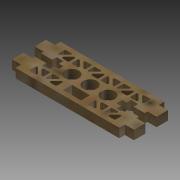
# Autodesk Inventor part: MotorCableHolder
Saved by Autodesk Inventor 2012 (Build 160160000, 160)
## iProperties
Created: 2014-07-20
Part Number: MotorCableHolder
Material: Default
Document SubType Name: Modeling
Designer: Anon
Density: 1 g/cm^3
Author: Anon
Autodesk Inventor part; units mm, degrees
ref_plane "YZ Plane" through (0, 0, 0) normal (1, 0, 0) x (0, 1, 0)
ref_plane "XZ Plane" through (0, 0, 0) normal (0, 1, 0) x (-1, 0, 0)
sketch "Sketch1" plane through (0, 0, 0) normal (0, 0, 1) x (1, 0, 0)
  line L0 (-27, 7.5) -> (-27, 2.5)
  line L1 (-27, 2.5) -> (-23, 2.5)
  line L2 (-27, 7.5) -> (-23, 7.5)
  line L3 (-23, 7.5) -> (-23, 10)
  line L4 (-23, 10) -> (0, 10)
  line L5 (0, 10) -> (0, 0)
  line L6 (0, 0) -> (-23, 0)
  line L7 (-23, 2.5) -> (-23, 0)
  line L8 (-27, -7.5) -> (-27, -2.5)
  line L9 (-27, -2.5) -> (-23, -2.5)
  line L10 (-27, -7.5) -> (-23, -7.5)
  line L11 (-23, -7.5) -> (-23, -10)
  line L12 (-23, -10) -> (0, -10)
  line L13 (0, -10) -> (0, 0)
  line L14 (-23, -2.5) -> (-23, 0)
  line L15 (27, 7.5) -> (27, 2.5)
  line L16 (27, 2.5) -> (23, 2.5)
  line L17 (27, 7.5) -> (23, 7.5)
  line L18 (23, 7.5) -> (23, 10)
  line L19 (23, 10) -> (0, 10)
  line L20 (0, 0) -> (23, 0)
  line L21 (23, 2.5) -> (23, 0)
  line L22 (27, -7.5) -> (27, -2.5)
  line L23 (27, -2.5) -> (23, -2.5)
  line L24 (27, -7.5) -> (23, -7.5)
  line L25 (23, -7.5) -> (23, -10)
  line L26 (23, -10) -> (0, -10)
  line L27 (23, -2.5) -> (23, 0)
  dimension "d0" = 5
  dimension "d1" = 4
  dimension "d12" = 27
  dimension "d13" = 4
  dimension "d14" = 2.5
  dimension "d53" = 2.5
  constraints: 56 end point, 17 symmetric about line, 3 perpendicular, 2 parallel, 1 vertical
  measures "d0" distance of L0.start L0.end
  measures "d1" distance of L0.end L1.end
  measures "d12" distance from line of L5.end L0
  measures "d13" distance of L0.start L2.end
  measures "d14" distance of L2.end L3.end
  measures "d53" distance of L1.end L6.end
extrude "Base" add sketch "Sketch1" along normal blind 4
sketch "Sketch2" plane through (0, 0, 4) normal (0, 0, 1) x (1, 0, 0)
  line L0 (-23, -2.5) -> (-23, 2.5) projected
  line L1 (-23, -10) -> (-23, -7.5) projected
  line L2 (-23, 1.25) -> (-18, 1.25)
  line L3 (-18, 1.25) -> (-18, 3.25)
  line L4 (-18, 3.25) -> (-15, 3.25)
  line L5 (-15, 3.25) -> (-15, 1.25)
  line L6 (-15, 1.25) -> (-13, 1.25)
  line L7 (-13, 1.25) -> (-13, -1.25)
  line L8 (-13, -1.25) -> (-15, -1.25)
  line L9 (-15, -1.25) -> (-15, -3.25)
  line L10 (-15, -3.25) -> (-18, -3.25)
  line L11 (-18, -3.25) -> (-18, -1.3408)
  line L12 (-18, -1.3408) -> (-23, -1.3408)
  line L13 (-23, 1.25) -> (-23, -1.3408)
  point P0 (0, 0)
  dimension "d17" = 5
  dimension "d18" = 2
  dimension "d19" = 3
  dimension "d20" = 2
  dimension "d21" = 2.5
  dimension "d22" = 2
  dimension "d23" = 1.25
  constraints: 24 end point, 6 parallel, 4 perpendicular, 2 collinear, 2 point on line
  measures "d17" distance of L2.start L2.end
  measures "d18" distance of L2.end L3.end
  measures "d19" distance of L3.end L4.end
  measures "d20" distance of L5.end L6.end
  measures "d21" distance of L6.end L7.end
  measures "d22" distance of L8.end L9.end
  measures "d23" distance from line of L2 point (0, 0)
extrude "ScrewLock" cut sketch "Sketch2" against normal blind 4
mirror "ScrewLockDoubler" about plane through (0, 0, 0) normal (1, 0, 0) of "ScrewLock"
sketch "Sketch3" plane through (0, 0, 4) normal (0, 0, 1) x (1, 0, 0)
  line L0 (18, 3.25) -> (18, 1.25) projected
  line L1 (-19, 8) -> (-19, 4)
  line L2 (-15, 8) -> (-19, 8)
  line L3 (-19, 4) -> (-15, 8)
  line L4 (-17.5, 4) -> (-13.5, 4)
  line L5 (-13.5, 4) -> (-13.5, 8)
  line L6 (-23, 10) -> (23, 10) projected
  line L7 (-23, 7.5) -> (-23, 10) projected
  line L8 (-13.5, 8) -> (-17.5, 4)
  point P0 (0, 0)
  dimension "d26" = 4
  dimension "d28" = 4
  dimension "d29" = 1.5
  dimension "d37" = 4
  dimension "d38" = 2
  dimension "d39" = 4
  constraints: 12 end point, 3 parallel, 2 perpendicular
  measures "d26" distance of L1.start L1.end
  measures "d28" distance of L4.start L4.end
  measures "d29" distance of L5.end L2.start
  measures "d37" distance between parallel lines of L7 L1
  measures "d38" distance between parallel lines of L6 L2
  measures "d39" distance of L4.end L5.end
extrude "FillPattern" cut sketch "Sketch3" against normal blind 4
fillet "FillPatternFillet" radius 0.5 6 edges at (-19, 8, 2) (-13.5, 4, 2) (-19, 4, 2) (-17.5, 4, 2) (-13.5, 8, 2) (-15, 8, 2)
ref_plane "PatternMirror" through (-13, 4.5, 4) normal (-1, 0, 0) x (0, 0, 1)
mirror "PatternSquare" about plane through (-13, 4.5, 4) normal (-1, 0, 0) of "FillPattern", "FillPatternFillet"
pattern_linear "TopSpread" count 3 spacing 13 along (1, 0, 0) of "FillPattern", "FillPatternFillet", "PatternSquare"
mirror "BottomSpread" about plane through (0, 0, 0) normal (0, 1, 0) of "FillPattern", "FillPatternFillet", "PatternSquare", "TopSpread"
sketch "Sketch4" plane through (0, 0, 4) normal (0, 0, 1) x (1, 0, 0)
  line L0 (18, 3.25) -> (18, 1.25) projected
  line L1 (0, 6.5) -> (0, -5) construction
  point P0 (0, 0)
  point P1 (0, 0)
  point P2 (-8, 0)
  point P3 (8, 0)
  dimension "d45" = 8
  constraints: 2 end point, 1 coincident, 1 parallel, 1 symmetric about line
  measures "d45" distance of point (0, 0) point (-8, 0)
hole "WireHoles" at (0, 0, 4) at (-8, 0, 4) at (8, 0, 4) direction (0, 0, -1) diameter 6 end through all
sketch "Sketch6" plane through (0, 0, 4) normal (0, 0, 1) x (1, 0, 0)
  line L0 (2.8536, -7.1464) -> (5.1464, -4.8536) projected
  arc A0 (6, -5.2071) -> (5.1464, -4.8536) centre (5.5, -5.2071) ccw projected
  line L1 (6, -5.2071) -> (6, -7.5) projected
  arc A1 (5.5, -8) -> (6, -7.5) centre (5.5, -7.5) ccw projected
  line L2 (5.5, -8) -> (3.2071, -8) projected
  arc A2 (2.8536, -7.1464) -> (3.2071, -8) centre (3.2071, -7.5) ccw projected
  line L3 (0.5, -6.7929) -> (0.5, -4.5) projected
  arc A3 (1, -4) -> (0.5, -4.5) centre (1, -4.5) ccw projected
  line L4 (1, -4) -> (3.2929, -4) projected
  arc A4 (3.6464, -4.8536) -> (3.2929, -4) centre (3.2929, -4.5) ccw projected
  line L5 (3.6464, -4.8536) -> (1.3536, -7.1464) projected
  arc A5 (0.5, -6.7929) -> (1.3536, -7.1464) centre (1, -6.7929) ccw projected
  line L6 (-5.1464, -4.8536) -> (-2.8536, -7.1464) projected
  arc A6 (-3.2071, -8) -> (-2.8536, -7.1464) centre (-3.2071, -7.5) ccw projected
  line L7 (-3.2071, -8) -> (-5.5, -8) projected
  arc A7 (-6, -7.5) -> (-5.5, -8) centre (-5.5, -7.5) ccw projected
  line L8 (-6, -7.5) -> (-6, -5.2071) projected
  arc A8 (-5.1464, -4.8536) -> (-6, -5.2071) centre (-5.5, -5.2071) ccw projected
  line L9 (-0.5, -4.5) -> (-0.5, -6.7929) projected
  arc A9 (-1.3536, -7.1464) -> (-0.5, -6.7929) centre (-1, -6.7929) ccw projected
  line L10 (-1.3536, -7.1464) -> (-3.6464, -4.8536) projected
  arc A10 (-3.2929, -4) -> (-3.6464, -4.8536) centre (-3.2929, -4.5) ccw projected
  line L11 (-3.2929, -4) -> (-1, -4) projected
  arc A11 (-0.5, -4.5) -> (-1, -4) centre (-1, -4.5) ccw projected
  line L12 (-6.3246, -3.6754) -> (6.5024, -3.6754)
  line L13 (6.5024, -3.6754) -> (6.5024, -8.75)
  line L14 (6.5024, -8.75) -> (-6.3246, -8.75)
  line L15 (-6.3246, -8.75) -> (-6.3246, -3.6754)
  constraints: 8 end point, 2 parallel, 1 horizontal, 1 perpendicular
extrude "BottomFiller" add sketch "Sketch6" against normal blind 4 contours L0 A0 L1 A1 L2 A2 | L3 A3 L4 A4 L5 A5 | L6 A6 L7 A7 L8 A8 | L9 A9 L10 A10 L11 A11
sketch "Sketch7" plane through (0, 0, 4) normal (0, 0, 1) x (1, 0, 0)
  circle A0 centre (0, 0) radius 3 projected
  line L0 (-4, -4) -> (4, -4)
  line L1 (4, -4) -> (4, -8)
  line L2 (4, -8) -> (-4, -8)
  line L3 (-4, -8) -> (-4, -4)
  dimension "d56" = 8
  dimension "d57" = 4
  dimension "d58" = 4
  dimension "d59" = 4
  constraints: 8 end point, 2 parallel, 1 horizontal, 1 perpendicular
  measures "d56" distance of L1.end L2.end
  measures "d57" distance of L0.end L1.end
  measures "d58" distance from line of A0.centre L3
  measures "d59" distance from line of L0 A0.centre
extrude "WingLedHole" cut sketch "Sketch7" against normal blind 4 contours L0 L1 L2 L3
body "Solid1"
